Spike (Autodesk Fusion 360 design; units mm, degrees)
Autodesk Fusion 360 part; units mm, degrees
sketch "Sketch1" plane through (0, 0, 0) normal (0, 0, 1) x (1, 0, 0)
  circle A0 centre (0, 125) radius 7.25
  circle A1 centre (0, 125) radius 11
  line L0 (-1, 0) -> (1, 0)
  line L1 (1, 0) -> (1, 125)
  line L2 (1, 125) -> (-1, 125)
  line L3 (-1, 125) -> (-1, 0)
  line L4 (-1, 0) -> (-6, 54.7723)
  line L5 (-6, 54.7723) -> (-1, 54.7723)
  line L6 (-6, 54.7723) -> (-6, 118.125)
  circle A2 centre (0, 125) radius 9.125
  line L7 (1, 0) -> (6, 54.7723)
  line L8 (6, 54.7723) -> (1, 54.7723)
  line L9 (6, 54.7723) -> (6, 118.125)
  point P0 (0, 125)
  point P1 (-36.2895, -2.8829)
  point P2 (0, 125)
  dimension "d10" = 14.5
  dimension "d11" = 22
  dimension "d32" = 2
  dimension "d33" = 125
  dimension "d34" = 55
  dimension "d35" = 5
  dimension "d37" = 18.25
  dimension "d38" = 55
  dimension "d40" = 5
  constraint coincident P2 P0
  constraint concentric A0 A1
  constraint horizontal L0
  constraint vertical L1
  constraint horizontal L2
  constraint vertical L3
  constraint coincident origin L0
  constraint midpoint origin L0
  constraint midpoint L2 P2
  constraint horizontal L5
  constraint coincident L3 L5.end
  constraint perpendicular L5 L6
  constraint concentric A1 A2
  constraint coincident L6.end A2
  constraint coincident L1 L8.end
  constraint perpendicular L1 L8
  constraint coincident A2 L9.end
  constraint perpendicular L8 L9
  measures "d10" diameter of A0
  measures "d11" diameter of A1
  measures "d32" distance of L0.start L0.end
  measures "d33" distance of L0.start L2.end
  measures "d34" distance of L0.start L4.end
  measures "d35" distance of L4.end L5.end
  measures "d37" diameter of A2
  measures "d38" distance of L0.end L7.end
  measures "d40" distance of L7.end L8.end
extrude "Extrude1" add sketch "Sketch1" along normal blind 2 contours A0 L1 L3 A2 | A0 L1 L3 A2 | A1 L1 L3 A2 | A1 L3 L6 A2 | A1 L1 A2 L9 | A1 L3 L5 L6 | A1 L0 L1 L3 | A1 L6 A2 L9 | A1 L1 L8 L9 | L3 L4 L5 | L1 L7 L8
sketch "Sketch4" plane through (0, 0, 0) normal (1, 0, 0) x (0, 1, 0)
  line L0 (0, 2) -> (54.7723, 7)
  line L1 (54.7723, 7) -> (54.7723, 2)
  line L2 (0, 2) -> (54.7723, 2)
  line L3 (116.5, 2) -> (116.5, 7)
  line L4 (54.7723, 7) -> (116.5, 7)
  line L5 (116.5, 2) -> (54.7723, 2)
  point P0 (0, 2)
  point P1 (0, 2)
  dimension "d42" = 55
  dimension "d43" = 5
  dimension "d44" = 5
  constraint coincident P0 L0.start
  constraint vertical L1
  constraint coincident L1.end L2
  constraint vertical L3
  measures "d42" distance of P1 L0.end
  measures "d43" distance of L0.end L1.end
  measures "d44" distance of L3.start L3.end
extrude "Extrude6" add sketch "Sketch4" along normal mid plane 2
extrude "Extrude4" add sketch "Sketch1" along normal blind 7 contours A0 L1 L3 A2 | A0 L1 L3 A2 | A1 L1 L3 A2 | A1 L3 L6 A2 | A1 L1 A2 L9 | A1 L6 A2 L9
sketch "Sketch2" plane through (0, 0, 7) normal (0, 0, 1) x (-1, 0, 0)
  circle A0 centre (6.3474, -130.27) radius 8.25
  line L0 (1, -114.0455) -> (1, -116.5)
  line L1 (1, -116.5) -> (-1, -116.5)
  line L2 (-1, -116.5) -> (-1, -114.0455)
  arc A1 (-1, -114.0455) -> (1, -114.0455) centre (0, -125) ccw
  circle A2 centre (0, -125) radius 7.25
  dimension "d16" = 16.5
  measures "d16" diameter of A0
extrude "Extrude3" cut sketch "Sketch2" against normal blind 20 contours A0 A1 | A0 A1 A2 | A0 A2 picked at (1.8654, -126.5575)
equation "d19 = blade + 2 mm"
equation "d35 = blade"
equation "d40 = blade"
equation "d43 = blade"
equation "d44 = blade"
equation "blade = 5 mm"
